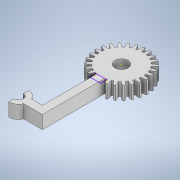
# Autodesk Inventor part: Free gear
Saved by Autodesk Inventor 2022 (Build 260153000, 153)
## iProperties
Created: 2022-02-25
Part Number: Free gear
Material: Generic
Document SubType Name: Modeling
Designer: Alexa
Density: 1 g/cm^3
Appearance: Default
Author: Alexa
Autodesk Inventor part; units mm, degrees
ref_plane "YZ Plane" through (0, 0, 0) normal (1, 0, 0) x (0, 1, 0)
ref_plane "XZ Plane" through (0, 0, 0) normal (0, 1, 0) x (-1, 0, 0)
ref_plane "XY Plane" through (0, 0, 0) normal (0, 0, 1) x (1, 0, 0)
sketch "Sketch1" plane through (0, 0, 0) normal (0, 1, 0) x (-1, 0, 0)
  circle A0 centre (0, 0) radius 8
  circle A1 centre (0, 0) radius 2
  line L0 (7.9113, 0.5933) -> (7.9113, -0.6067)
  line L1 (9.9113, -0.2567) -> (9.9113, 0.2433)
  line L2 (7.6237, -0.0067) -> (9.0479, -0.0067) construction
  arc A2 (9.9113, 0.2433) -> (7.9113, 0.5933) centre (8.1555, -3.9001) ccw construction
  arc A3 (7.9113, -0.6067) -> (9.9113, -0.2567) centre (8.1555, 3.8866) ccw construction
  arc A4 (9.9113, 0.2433) -> (7.9113, 0.5933) centre (8.1555, -3.9001) ccw construction
  arc A5 (9.9113, 0.2433) -> (7.9777, 0.5964) centre (8.1555, -3.9001) ccw
  arc A6 (7.9767, -0.6098) -> (9.9113, -0.2567) centre (8.1555, 3.8866) ccw
  line L3 (9.4, 0) -> (9.4, -0.4379)
  line L4 (9.4, 0) -> (9.4, 0.4244)
  arc A7 (5.296, -1.8919) -> (5.296, 1.8784) centre (4.6281, -0.0067) ccw
  circle A8 centre (0, 0) radius 8
  dimension "d0" = 16
  dimension "d1" = 4
  dimension "d2" = 0.25
  dimension "d3" = 0.25
  dimension "d4" = 0.6
  dimension "d7" = 1.2
  dimension "d8" = 4.5
  dimension "d10" = 2
  constraints: 18 point on circle, 10 end point, 9 centre point, 4 concentric, 3 coincident, 2 vertical, 1 horizontal, 1 parallel, 1 point on line
  measures "d0" diameter of A0
  measures "d1" diameter of A1
  measures "d2" distance from line of L1.start L2
  measures "d3" distance from line of L1.end L2
  measures "d4" distance from line of L0.start L2
  measures "d7" distance of L0.end L0.start
  measures "d8" radius of A3
  measures "d10" radius of A7
extrude "Extrusion1" add sketch "Sketch1" along normal blind 5
pattern_circular "Circular Pattern1" count 26 over 360 about axis through (0, 0, 0) along (0, 1, 0) of "Extrusion1"
sketch "Sketch8" plane through (0, 5, 0) normal (0, 1, 0) x (1, 0, 0)
  circle A0 centre (0, 0) radius 2.5
  circle A1 centre (0, 0) radius 2
  dimension "d49" = 5
  dimension "d50" = 4
  constraints: 2 centre point, 2 coincident
  measures "d49" diameter of A0
  measures "d50" diameter of A1
extrude "Extrusion6" cut sketch "Sketch8" against normal blind 13.8125
sketch "Sketch11" plane through (0, 5, 0) normal (0, 1, 0) x (1, 0, 0)
  line L0 (0, 0) -> (30, 0)
  line L1 (30, 0) -> (30, -9)
  line L2 (30, -9) -> (0, -9)
  line L3 (0, -9) -> (0, 0)
  circle A0 centre (30, -9) radius 1.75
  dimension "d84" = 30
  dimension "d85" = 9
  dimension "d86" = 3.5
  constraints: 8 end point, 2 parallel, 1 centre point, 1 coincident, 1 horizontal, 1 perpendicular
  measures "d84" distance of L1.end L2.end
  measures "d85" distance of L0.end L1.end
  measures "d86" diameter of A0
extrude "Extrusion9" cut sketch "Sketch11" against normal blind 10 contours A0 L2 L1 | L1 L2 A0
sketch "Sketch12" plane through (0, 5, 0) normal (0, 1, 0) x (1, 0, 0)
  circle A0 centre (0, 0) radius 2.5 projected
  line L0 (0, 0) -> (-1.5, 0)
  line L1 (-1.5, 0) -> (-1.5, -14.191)
  line L2 (-1.5, -14.191) -> (0, -14.191)
  line L3 (0, -14.191) -> (0, 0)
  line L4 (0, -14.191) -> (1.5, -14.191)
  line L5 (1.5, -14.191) -> (1.5, -6.1824)
  line L6 (1.5, -6.1824) -> (0, -6.1824)
  line L7 (0, -6.1824) -> (0, -14.191)
  line L8 (-1.5, -14.191) -> (0, -14.191)
  line L9 (0, -14.191) -> (0, -6.1824)
  line L10 (0, -6.1824) -> (-1.5, -6.1824)
  line L11 (-1.5, -6.1824) -> (-1.5, -14.191)
  dimension "d89" = 1.5
  dimension "d90" = 1.5
  constraints: 24 end point, 6 parallel, 3 horizontal, 3 perpendicular
  measures "d89" distance of L2.end L1.end
  measures "d90" distance of L6.end L5.end
extrude "Extrusion10" cut sketch "Sketch12" against normal blind 10 contours L10 L3 L2 L1 | L6 L5 L4 L3
sketch "Sketch13" plane through (0, 5, 0) normal (0, 1, 0) x (1, 0, 0)
  arc A0 (-1.5669, -7.8451) -> (-1.5, -9.6168) centre (2.8753, -8.5646) ccw projected
  line L0 (1.5537, -7.8477) -> (-1.5669, -7.8451)
  line L1 (2.1693, -7.8482) -> (-2.0082, -7.8482)
  line L2 (-2.0082, -7.8482) -> (-2.0082, -10.2143)
  line L3 (-2.0082, -10.2143) -> (2.1693, -10.2143)
  line L4 (2.1693, -10.2143) -> (2.1693, -7.8482)
  point P0 (0, 0)
  constraints: 10 end point, 2 parallel, 1 horizontal, 1 perpendicular
sketch "Sketch14" plane through (0, 5, 0) normal (0, 1, 0) x (1, 0, 0)
  line L0 (1.9129, -7.8477) -> (1.156, -7.8477)
  line L1 (1.156, -7.8477) -> (1.156, -9.6618)
  line L2 (1.156, -9.6618) -> (1.9129, -9.6618)
  line L3 (1.9129, -9.6618) -> (1.9129, -7.8477)
  line L4 (1.156, -9.6618) -> (-2.0763, -9.6618)
  line L5 (-2.0763, -9.6618) -> (-2.0763, -7.8477)
  line L6 (-2.0763, -7.8477) -> (1.156, -7.8477)
  line L7 (1.156, -7.8477) -> (1.156, -9.6618)
  point P0 (0, 0)
  constraints: 16 end point, 4 parallel, 2 horizontal, 2 perpendicular, 1 point on line
extrude "Extrusion11" cut sketch "Sketch14" against normal blind 10
sketch "Sketch15" plane through (0, 5, 0) normal (0, 1, 0) x (1, 0, 0)
  line L0 (0, 0) -> (-9, 0)
  line L1 (-9, 0) -> (-9, -30)
  line L2 (-9, -30) -> (0, -30)
  line L3 (0, -30) -> (0, 0)
  line L4 (1.5, -6.1824) -> (1.5, -7.8477) projected
  line L5 (1.5, -6.1824) -> (-1.5, -6.1824)
  line L6 (-1.5, -6.1824) -> (-1.5, -30)
  line L7 (-1.5, -30) -> (1.5, -30)
  line L8 (1.5, -30) -> (1.5, -6.1824)
  line L9 (1.5, -30) -> (-9, -30)
  line L10 (-9, -30) -> (-9, -31.5)
  line L11 (-9, -31.5) -> (1.5, -31.5)
  line L12 (1.5, -31.5) -> (1.5, -30)
  line L13 (1.5, -30) -> (-9, -30)
  line L14 (-9, -30) -> (-9, -28.5)
  line L15 (-9, -28.5) -> (1.5, -28.5)
  line L16 (1.5, -28.5) -> (1.5, -30)
  circle A0 centre (-9, -30) radius 1.75
  circle A1 centre (-9, -30) radius 2.5
  line L17 (-9, -31.5) -> (-9, -32.8448)
  line L18 (-9, -32.8448) -> (-9, -26.54)
  point P0 (-1.5, -28.5)
  point P1 (-7, -28.5)
  point P2 (-9, -27.5)
  point P3 (-9, -28.25)
  point P4 (-9, -31.75)
  point P5 (-9, -32.5)
  point P6 (-7, -31.5)
  dimension "d95" = 9
  dimension "d96" = 30
  dimension "d97" = 3
  dimension "d98" = 1.5
  dimension "d99" = 1.5
  dimension "d100" = 3.5
  dimension "d101" = 5
  constraints: 36 end point, 8 parallel, 5 perpendicular, 4 horizontal, 4 point on line, 2 centre point, 2 coincident
  measures "d95" distance of L2.end L1.end
  measures "d96" distance of L1.end L0.end
  measures "d97" distance of L7.end L6.end
  measures "d98" distance of L10.end L9.end
  measures "d99" distance of L13.end L14.end
  measures "d100" diameter of A0
  measures "d101" diameter of A1
extrude "Extrusion12" add sketch "Sketch15" against normal blind 5 contours L5 L4 L8 L15 L3 | L3 L15 L6 L5 | L15 L8 L7 L3 | L3 L2 L6 L15 | A1 L15 A0 L1 | L7 L12 L11 A1 L2 | L6 L2 A1 L15 | A1 L2 A0 L15 | L17 A0 L11 A1 | A1 L11 A0 L2
sketch "Sketch16" plane through (0, 5, 0) normal (0, 1, 0) x (1, 0, 0)
  arc A0 (-9, -31.75) -> (-9, -28.25) centre (-9, -30) ccw projected
  circle A1 centre (-9, -30) radius 1.75
  line L0 (-9, -31.75) -> (-9, -33.75)
  line L1 (-9, -28.25) -> (-9, -27.5) projected
  line L2 (-9, -28.25) -> (-9, -26.25)
  circle A2 centre (-9, -30) radius 3.75
  circle A3 centre (-9, -30) radius 2.5
  line L3 (1.5, -31.5) -> (-7, -31.5) projected
  line L4 (-5.5631, -31.5) -> (-7, -31.5)
  line L5 (-1.5, -28.5) -> (-7, -28.5) projected
  line L6 (-5.5631, -28.5) -> (-7, -28.5)
  point P0 (0, 0)
  point P1 (-9, -32.5)
  dimension "d104" = 2
  dimension "d105" = 2
  dimension "d106" = 7.5
  dimension "d107" = 5
  constraints: 8 end point, 3 centre point, 3 coincident, 2 collinear, 2 point on circle, 2 point on line, 2 vertical
  measures "d104" distance of L0.start L0.end
  measures "d105" distance of L1.start L2.end
  measures "d106" diameter of A2
  measures "d107" diameter of A3
extrude "Extrusion13" add sketch "Sketch16" against normal blind 5 contours A3 L3 A2 L0 | L2 A2 L5 A3
body "Solid1"
